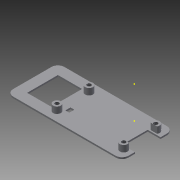
# Autodesk Inventor part: Case Relay
Saved by Autodesk Inventor 2015 (Build 190159000, 159)
## iProperties
Created: 2017-12-18
Part Number: Case Relay
Material: Generic
Document SubType Name: Modeling
Designer: Toby
Density: 1 g/cm^3
Appearance: Default
Author: Toby
Autodesk Inventor part; units mm, degrees
ref_plane "YZ Plane" through (0, 0, 0) normal (1, 0, 0) x (0, 1, 0)
ref_plane "XZ Plane" through (0, 0, 0) normal (0, 1, 0) x (-1, 0, 0)
ref_plane "XY Plane" through (0, 0, 0) normal (0, 0, 1) x (1, 0, 0)
sketch "Sketch1" plane through (0, 0, 0) normal (0, 0, 1) x (1, 0, 0)
  line L0 (-66.7657, 11.6667) -> (16.2343, 11.6667)
  line L1 (16.2343, 11.6667) -> (16.2343, -23.3333)
  line L2 (16.2343, -23.3333) -> (-66.7657, -23.3333)
  line L3 (-66.7657, -23.3333) -> (-66.7657, 11.6667)
  point P0 (0, 0)
  dimension "d0" = 35
  dimension "d1" = 83
  constraints: 8 end point, 2 parallel, 1 horizontal, 1 perpendicular
  measures "d0" distance of L2.end L0.start
  measures "d1" distance of L0.start L0.end
extrude "Extrusion1" add sketch "Sketch1" along normal blind 1.2
sketch "Sketch2" plane through (0, 0, 1.2) normal (0, 0, 1) x (1, 0, 0)
  line L0 (16.2343, -23.3333) -> (16.2343, 11.6667) projected
  line L1 (-66.7657, 11.6667) -> (16.2343, 11.6667)
  line L2 (16.2343, 11.6667) -> (16.2343, 9.8667)
  line L3 (16.2343, 9.8667) -> (-66.7657, 9.8667)
  line L4 (-66.7657, 9.8667) -> (-66.7657, 11.6667)
  line L5 (-66.7657, 11.6667) -> (-66.7657, -23.3333) projected
  line L6 (16.2343, -23.3333) -> (-66.7657, -23.3333)
  line L7 (-66.7657, -23.3333) -> (-66.7657, -21.5333)
  line L8 (-66.7657, -21.5333) -> (16.2343, -21.5333)
  line L9 (16.2343, -21.5333) -> (16.2343, -23.3333)
  line L10 (-66.7657, 9.8667) -> (-65.5657, 9.8667)
  line L11 (-65.5657, 9.8667) -> (-65.5657, -21.5333)
  line L12 (-65.5657, -21.5333) -> (-66.7657, -21.5333)
  line L13 (-66.7657, -21.5333) -> (-66.7657, 9.8667)
  line L14 (16.2343, 9.8667) -> (15.0343, 9.8667)
  line L15 (15.0343, 9.8667) -> (15.0343, -21.5333)
  line L16 (15.0343, -21.5333) -> (16.2343, -21.5333)
  line L17 (16.2343, -21.5333) -> (16.2343, 9.8667)
  line L18 (-66.7657, 11.6667) -> (-65.5657, 11.6667)
  line L19 (-65.5657, 11.6667) -> (-65.5657, -21.5333)
  line L20 (-65.5657, -21.5333) -> (-66.7657, -21.5333)
  line L21 (-66.7657, -21.5333) -> (-66.7657, 11.6667)
  line L22 (-66.7657, 11.6667) -> (16.2343, 11.6667)
  line L23 (16.2343, 11.6667) -> (16.2343, 9.8667)
  line L24 (16.2343, 9.8667) -> (-66.7657, 9.8667)
  line L25 (-66.7657, 9.8667) -> (-66.7657, 11.6667)
  point P0 (0, 0)
  dimension "d4" = 1.8
  dimension "d5" = 1.8
  dimension "d6" = 1.2
  dimension "d7" = 1.2
  constraints: 48 end point, 12 parallel, 6 horizontal, 6 perpendicular, 4 point on line
  measures "d4" distance between parallel lines of L1 L3
  measures "d5" distance between parallel lines of L6 L8
  measures "d6" distance between parallel lines of L13 L11
  measures "d7" distance between parallel lines of L17 L15
extrude "Extrusion2" add sketch "Sketch2" along normal blind 30 contours L6 L5 L8 L0 | L8 L15 L3 L0 | L3 L19 L1 L0 | L5 L3 L11 L8 | L4 L1 L19 L3
sketch "Sketch3" plane through (0, 0, 31.2) normal (0, 0, 1) x (1, 0, 0)
  point P0 (0, 0)
sketch "Sketch4" plane through (16.2343, -23.3333, 0) normal (1, 0, 0) x (0, 0, -1)
  line L0 (-1.2, 33.2) -> (-1.2, 1.8) projected
  line L1 (-1.2, 7.5) -> (-6.2, 7.5)
  line L2 (-6.2, 7.5) -> (-6.2, 27.5)
  line L3 (-6.2, 27.5) -> (-1.2, 27.5)
  line L4 (-1.2, 27.5) -> (-1.2, 7.5)
  line L5 (-1.2, 1.8) -> (-31.2, 1.8) projected
  line L6 (-1.2, 33.2) -> (-31.2, 33.2) projected
  line L7 (-6.2, 7.5) -> (0, 7.5)
  line L8 (0, 7.5) -> (0, 27.5)
  line L9 (0, 27.5) -> (-6.2, 27.5)
  line L10 (-6.2, 27.5) -> (-6.2, 7.5)
  line L11 (0, 35) -> (0, 0) projected
  point P0 (0, 23.3333)
  dimension "d10" = 20
  dimension "d11" = 5
  dimension "d12" = 5.7
  dimension "d13" = 5.7
  constraints: 16 end point, 4 parallel, 2 collinear, 2 horizontal, 2 perpendicular, 1 point on line
  measures "d10" distance of L1.end L2.end
  measures "d11" distance between parallel lines of L2 L0
  measures "d12" distance between parallel lines of L5 L1
  measures "d13" distance between parallel lines of L6 L3
extrude "Extrusion3" cut sketch "Sketch4" against normal blind 10
fillet "Fillet1" radius 2 8 edges at (-66.7657, 11.6667, 15.6) (-65.5657, 9.8667, 16.2) (-66.7657, -23.3333, 15.6) (-65.5657, -21.5333, 16.2) (15.0343, 9.8667, 16.2) (16.2343, 11.6667, 15.6) (16.2343, -23.3333, 15.6) (15.0343, -21.5333, 16.2)
sketch "Sketch5" plane through (0, 0, 1.2) normal (0, 0, 1) x (1, 0, 0)
  circle A0 centre (10.0343, 6.6667) radius 1.5
  circle A1 centre (10.0343, -18.3333) radius 1.5
  line L0 (15.0343, 7.8667) -> (15.0343, -19.5333) projected
  line L1 (13.0343, -21.5333) -> (-63.5657, -21.5333) projected
  line L2 (-63.5657, 9.8667) -> (13.0343, 9.8667) projected
  point P0 (0, 0)
  dimension "d17" = 3
  dimension "d18" = 3
  dimension "d19" = 25
  dimension "d20" = 5
  dimension "d21" = 5
  dimension "d22" = 3.2
  dimension "d23" = 3.2
  constraints: 2 centre point
  measures "d17" diameter of A0
  measures "d18" diameter of A1
  measures "d19" distance of A1.centre A0.centre
  measures "d20" distance from line of L0 A0.centre
  measures "d21" distance from line of L0 A1.centre
  measures "d22" distance from line of L1 A1.centre
  measures "d23" distance from line of L2 A0.centre
extrude "Extrusion4" add sketch "Sketch5" along normal blind 5
sketch "Sketch6" plane through (0, 0, 1.2) normal (0, 0, 1) x (1, 0, 0)
  circle A0 centre (-41.9656, -18.3962) radius 1.5
  circle A1 centre (-41.9656, 6.6038) radius 1.5
  circle A2 centre (10.0343, 6.6667) radius 1.5 projected
  circle A3 centre (10.0343, -18.3333) radius 1.5 projected
  point P0 (0, 0)
  dimension "d26" = 3
  dimension "d27" = 3
  dimension "d28" = 25
  dimension "d29" = 52
  dimension "d30" = 52
  constraints: 2 centre point
  measures "d26" diameter of A0
  measures "d27" diameter of A1
  measures "d28" distance of A1.centre A0.centre
  measures "d29" distance of A2.centre A1.centre
  measures "d30" distance of A3.centre A0.centre
extrude "Extrusion5" add sketch "Sketch6" along normal blind 5 contours A0 | A1
sketch "Sketch7" plane through (-41.9656, 6.6038, 6.2) normal (0, 0, 1) x (1, 0, 0)
  point P0 (41.9656, -6.6038)
sketch "Sketch8" plane through (0, 0, 1.2) normal (0, 0, 1) x (1, 0, 0)
  circle A0 centre (-41.9656, -18.3962) radius 1.5 projected
  circle A1 centre (-41.9656, -18.3962) radius 3
  circle A2 centre (-41.9656, 6.6038) radius 1.5 projected
  circle A3 centre (-41.9656, 6.6038) radius 3
  circle A4 centre (10.0343, -18.3333) radius 1.5 projected
  circle A5 centre (10.0343, -18.3333) radius 3
  circle A6 centre (10.0343, 6.6667) radius 1.5 projected
  circle A7 centre (10.0343, 6.6667) radius 3
  point P0 (0, 0)
  dimension "d33" = 6
  dimension "d34" = 6
  dimension "d35" = 6
  dimension "d36" = 6
  constraints: 4 centre point, 4 coincident
  measures "d33" diameter of A1
  measures "d34" diameter of A3
  measures "d35" diameter of A7
  measures "d36" diameter of A5
extrude "Extrusion6" add sketch "Sketch8" along normal blind 5
sketch "Sketch9" plane through (0, 0, 1.2) normal (0, 0, 1) x (1, 0, 0)
  arc A0 (8.376, -15.8333) -> (11.6926, -15.8333) centre (10.0343, -18.3333) ccw projected
  circle A1 centre (10.0343, -18.3333) radius 3
  arc A2 (11.6926, 4.1667) -> (8.376, 4.1667) centre (10.0343, 6.6667) ccw projected
  circle A3 centre (10.0343, 6.6667) radius 3
  point P0 (0, 0)
  dimension "d39" = 6
  dimension "d40" = 6
  constraints: 2 centre point, 2 coincident
  measures "d39" diameter of A1
  measures "d40" diameter of A3
extrude "Extrusion7" add sketch "Sketch9" against normal blind 1.2
sketch "Sketch10" plane through (-41.9656, -18.3962, 6.2) normal (0, 0, 1) x (1, 0, 0)
  circle A0 centre (0, 0) radius 3 projected
  circle A1 centre (0, 0) radius 1.5
  circle A2 centre (0, 25) radius 3 projected
  circle A3 centre (0, 25) radius 1.5
  circle A4 centre (52, 0.0629) radius 3 projected
  circle A5 centre (52, 0.0629) radius 1.5
  circle A6 centre (52, 25.0629) radius 3 projected
  circle A7 centre (52, 25.0629) radius 1.5
  point P0 (41.9656, 18.3962)
  dimension "d43" = 3
  dimension "d44" = 3
  dimension "d45" = 3
  dimension "d46" = 3
  constraints: 4 centre point, 4 coincident
  measures "d43" diameter of A1
  measures "d44" diameter of A3
  measures "d45" diameter of A5
  measures "d46" diameter of A7
extrude "Extrusion8" cut sketch "Sketch10" against normal blind 4 contours A1 | A3 | A5 | A7
thread "Thread1" size "M3x0.5" class "6H" standard "ANSI Metric M Profile" full length
thread "Thread2" size "M3x0.5" class "6H" standard "ANSI Metric M Profile" full length
thread "Thread3" size "M3x0.5" class "6H" standard "ANSI Metric M Profile" full length
thread "Thread4" size "M3x0.5" class "6H" standard "ANSI Metric M Profile" full length
sketch "Sketch11" plane through (0, 0, 31.2) normal (0, 0, 1) x (1, 0, 0)
  arc A0 (-64.7657, 11.6667) -> (-66.7657, 9.6667) centre (-64.7657, 9.6667) ccw projected
  line L0 (-66.7657, 9.6667) -> (16.2343, 9.6667)
  line L1 (16.2343, 9.6667) -> (16.2343, 14.6667)
  line L2 (16.2343, 14.6667) -> (-66.7657, 14.6667)
  line L3 (-66.7657, 14.6667) -> (-66.7657, 9.6667)
  line L4 (16.2343, -21.3333) -> (-66.7657, -21.3333)
  line L5 (-66.7657, -21.3333) -> (-66.7657, -26.3333)
  line L6 (-66.7657, -26.3333) -> (16.2343, -26.3333)
  line L7 (16.2343, -26.3333) -> (16.2343, -21.3333)
  point P0 (0, 0)
  dimension "d57" = 5
  dimension "d58" = 5
  dimension "d59" = 83
  constraints: 16 end point, 4 parallel, 2 horizontal, 2 perpendicular, 1 point on circle, 1 point on line
  measures "d57" distance of L1.end L0.end
  measures "d58" distance of L5.end L4.end
  measures "d59" distance between parallel lines of L3 L1
extrude "Extrusion9" add sketch "Sketch11" against normal blind 31.2
fillet "Fillet2" radius 2 4 edges at (16.2343, -26.3333, 15.6) (16.2343, 14.6667, 15.6) (-66.7657, 14.6667, 15.6) (-66.7657, -26.3333, 15.6)
sketch "Sketch12" plane through (0, 0, 31.2) normal (0, 0, 1) x (1, 0, 0)
  line L0 (14.2343, -26.3333) -> (-64.7657, -26.3333) projected
  line L1 (8.2343, -26.3333) -> (-58.7657, -26.3333)
  line L2 (-58.7657, -26.3333) -> (-58.7657, -23.1333)
  line L3 (-58.7657, -23.1333) -> (8.2343, -23.1333)
  line L4 (8.2343, -23.1333) -> (8.2343, -26.3333)
  line L5 (-64.7657, 14.6667) -> (14.2343, 14.6667) projected
  line L6 (8.2343, 14.6667) -> (-58.7657, 14.6667)
  line L7 (-58.7657, 14.6667) -> (-58.7657, 11.4667)
  line L8 (-58.7657, 11.4667) -> (8.2343, 11.4667)
  line L9 (8.2343, 11.4667) -> (8.2343, 14.6667)
  line L10 (16.2343, -24.3333) -> (16.2343, 12.6667) projected
  line L11 (-66.7657, 12.6667) -> (-66.7657, -24.3333) projected
  line L12 (13.9061, -21.3333) -> (-64.4375, -21.3333) projected
  line L13 (10.0343, 9.6667) -> (-64.4375, 9.6667) projected
  point P0 (0, 0)
  dimension "d63" = 8
  dimension "d64" = 8
  dimension "d65" = 1.8
  dimension "d66" = 1.8
  constraints: 16 end point, 4 parallel, 4 point on line, 2 horizontal, 2 perpendicular
  measures "d63" distance between parallel lines of L10 L4
  measures "d64" distance between parallel lines of L11 L2
  measures "d65" distance between parallel lines of L12 L3
  measures "d66" distance between parallel lines of L13 L8
extrude "Extrusion10" cut sketch "Sketch12" against normal blind 31.2
fillet "Fillet3" radius 2 4 edges at (8.2343, -26.3333, 15.6) (-58.7657, -26.3333, 15.6) (8.2343, 14.6667, 15.6) (-58.7657, 14.6667, 15.6)
sketch "Sketch13" plane through (0, 0, 31.2) normal (0, 0, 1) x (1, 0, 0)
  line L0 (14.2343, -26.3333) -> (10.2343, -26.3333) projected
  circle A0 centre (12.2343, -23.9333) radius 1.5
  circle A1 centre (-62.7657, -23.9333) radius 1.5
  line L1 (-64.7657, -26.3333) -> (-60.7657, -26.3333) projected
  circle A2 centre (12.2343, 12.2667) radius 1.5
  circle A3 centre (-62.7657, 12.2667) radius 1.5
  line L2 (-66.7657, 12.6667) -> (-66.7657, -24.3333) projected
  line L3 (-60.7657, 14.6667) -> (-64.7657, 14.6667) projected
  line L4 (16.2343, -24.3333) -> (16.2343, 12.6667) projected
  line L5 (14.2343, 14.6667) -> (10.2343, 14.6667) projected
  line L6 (8.2343, -23.1333) -> (8.2343, -24.3333) projected
  point P0 (0, 0)
  dimension "d70" = 2.4
  dimension "d71" = 3
  dimension "d72" = 3
  dimension "d73" = 2.4
  dimension "d74" = 3
  dimension "d75" = 3
  dimension "d76" = 4
  dimension "d77" = 4
  dimension "d78" = 2.4
  dimension "d79" = 4
  dimension "d80" = 2.4
  dimension "d81" = 4
  constraints: 4 centre point, 1 coincident
  measures "d70" distance from line of L0 point (12.234, -23.933)
  measures "d71" diameter of A0
  measures "d72" diameter of A1
  measures "d73" distance from line of A1.centre L1
  measures "d74" diameter of A2
  measures "d75" diameter of A3
  measures "d76" distance from line of L2 A1.centre
  measures "d77" distance from line of L2 A3.centre
  measures "d78" distance from line of L3 A3.centre
  measures "d79" distance from line of L4 A2.centre
  measures "d80" distance from line of L5 A2.centre
  measures "d81" distance from line of L6 A0.centre
hole "Hole1" at (12.2343, -23.9333, 31.2) at (12.2343, 12.2667, 31.2) at (-62.7657, -23.9333, 31.2) at (-62.7657, 12.2667, 31.2) direction (0, 0, -1) diameter 3 depth 5 tip angle 118
sketch "Sketch14" plane through (0, 0, 31.2) normal (0, 0, 1) x (1, 0, 0)
  line L0 (-68.9331, 15.611) -> (20.031, 15.611)
  line L1 (20.031, 15.611) -> (20.031, -27.6485)
  line L2 (20.031, -27.6485) -> (-68.9331, -27.6485)
  line L3 (-68.9331, -27.6485) -> (-68.9331, 15.611)
  point P0 (0, 0)
  constraints: 8 end point, 2 parallel, 1 horizontal, 1 perpendicular
extrude "Extrusion11" cut sketch "Sketch14" against normal blind 25
sketch "Sketch15" plane through (0, 0, 6.2) normal (0, 0, 1) x (1, 0, 0)
  line L0 (-73.259, 21.6297) -> (22.194, 21.6297)
  line L1 (22.194, 21.6297) -> (22.194, 9.6667)
  line L2 (22.194, 9.6667) -> (-73.259, 9.6667)
  line L3 (-73.259, 9.6667) -> (-73.259, 21.6297)
  line L4 (-69.8735, -21.3333) -> (26.0497, -21.3333)
  line L5 (26.0497, -21.3333) -> (26.0497, -30.3757)
  line L6 (26.0497, -30.3757) -> (-69.8735, -30.3757)
  line L7 (-69.8735, -30.3757) -> (-69.8735, -21.3333)
  line L8 (10.0343, 9.6667) -> (-64.4375, 9.6667) projected
  line L9 (-41.3548, -21.3333) -> (10.0343, -21.3333) projected
  point P0 (0, 0)
  constraints: 16 end point, 4 parallel, 2 collinear, 2 horizontal, 2 perpendicular
extrude "Extrusion12" cut sketch "Sketch15" against normal blind 25
sketch "Sketch16" plane through (0, 0, 1.2) normal (0, 0, 1) x (1, 0, 0)
  line L0 (6.2343, 4.1667) -> (16.2343, 4.1667)
  line L1 (16.2343, 4.1667) -> (16.2343, -15.8333)
  line L2 (16.2343, -15.8333) -> (6.2343, -15.8333)
  line L3 (6.2343, -15.8333) -> (6.2343, 4.1667)
  point P0 (0, 0)
  constraints: 8 end point, 2 parallel, 1 horizontal, 1 perpendicular
extrude "Extrusion13" cut sketch "Sketch16" against normal blind 25
sketch "Sketch17" plane through (0, 0, 1.2) normal (0, 0, 1) x (1, 0, 0)
  line L0 (6.2343, 4.1667) -> (16.2343, 4.1667)
  line L1 (16.2343, 4.1667) -> (16.2343, -15.8333)
  line L2 (16.2343, -15.8333) -> (6.2343, -15.8333)
  line L3 (6.2343, -15.8333) -> (6.2343, 4.1667)
  point P0 (0, 0)
  constraints: 8 end point, 2 parallel, 1 horizontal, 1 perpendicular
extrude "Extrusion14" cut sketch "Sketch17" along normal blind 25
sketch "Sketch18" plane through (0, 0, 1.2) normal (0, 0, 1) x (1, 0, 0)
  line L0 (15.0343, -19.5333) -> (15.0343, -15.8333) projected
  line L1 (6.2343, 5.1667) -> (15.0343, 5.1667)
  line L2 (15.0343, 5.1667) -> (15.0343, -16.8333)
  line L3 (15.0343, -16.8333) -> (6.2343, -16.8333)
  line L4 (6.2343, -16.8333) -> (6.2343, 5.1667)
  line L5 (6.2343, 4.1667) -> (8.376, 4.1667) projected
  line L6 (15.0343, -15.8333) -> (11.6926, -15.8333) projected
  line L7 (6.2343, -15.8333) -> (6.2343, 4.1667) projected
  point P0 (0, 0)
  dimension "d97" = 1
  dimension "d98" = 1
  constraints: 8 end point, 2 parallel, 1 collinear, 1 horizontal, 1 perpendicular, 1 point on line
  measures "d97" distance between parallel lines of L5 L1
  measures "d98" distance between parallel lines of L6 L3
extrude "Extrusion15" cut sketch "Sketch18" along normal blind 25
sketch "Sketch19" plane through (0, 0, 6.2) normal (0, 0, 1) x (1, 0, 0)
  line L0 (13.9061, 9.6667) -> (16.2343, 9.6667)
  line L1 (16.2343, 9.6667) -> (16.2343, -21.3333)
  line L2 (16.2343, -21.3333) -> (13.9061, -21.3333)
  line L3 (13.9061, -21.3333) -> (13.9061, 9.6667)
  line L4 (-66.7657, 9.6667) -> (-64.4375, 9.6667)
  line L5 (-64.4375, 9.6667) -> (-64.4375, -21.3333)
  line L6 (-64.4375, -21.3333) -> (-66.7657, -21.3333)
  line L7 (-66.7657, -21.3333) -> (-66.7657, 9.6667)
  point P0 (0, 0)
  constraints: 16 end point, 4 parallel, 2 horizontal, 2 perpendicular
extrude "Extrusion16" cut sketch "Sketch19" against normal blind 5
sketch "Sketch20" plane through (0, 0, 1.2) normal (0, 0, 1) x (1, 0, 0)
  line L0 (-73.7657, 14.1667) -> (16.2343, 14.1667)
  line L1 (16.2343, 14.1667) -> (16.2343, -25.8333)
  line L2 (16.2343, -25.8333) -> (-73.7657, -25.8333)
  line L3 (-73.7657, -25.8333) -> (-73.7657, 14.1667)
  line L4 (16.2343, 9.6667) -> (16.2343, 4.1667) projected
  line L5 (-66.7657, 9.6667) -> (16.2343, 9.6667) projected
  line L6 (-41.3548, -21.3333) -> (10.0343, -21.3333) projected
  line L7 (-66.7657, -21.3333) -> (-66.7657, 9.6667) projected
  line L8 (16.2343, 4.1667) -> (6.2343, 4.1667)
  line L9 (6.2343, 4.1667) -> (6.2343, -15.8333)
  line L10 (6.2343, -15.8333) -> (16.2343, -15.8333)
  line L11 (16.2343, -15.8333) -> (16.2343, 4.1667)
  point P0 (0, 0)
  dimension "d103" = 90
  dimension "d104" = 40
  dimension "d105" = 4.5
  dimension "d106" = 4.5
  dimension "d107" = 7
  constraints: 16 end point, 4 parallel, 2 horizontal, 2 perpendicular, 1 collinear
  measures "d103" distance between parallel lines of L1 L3
  measures "d104" distance between parallel lines of L2 L0
  measures "d105" distance between parallel lines of L5 L0
  measures "d106" distance between parallel lines of L2 L6
  measures "d107" distance between parallel lines of L3 L7
extrude "Extrusion17" add sketch "Sketch20" against normal blind 1.2 contours L0 L1 L8 L9 L10 L2 L3
fillet "Fillet4" radius 5 4 edges at (-73.7657, 14.1667, 0.6) (-73.7657, -25.8333, 0.6) (16.2343, -25.8333, 0.6) (16.2343, 14.1667, 0.6)
sketch "Sketch21" plane through (0, 0, 1.2) normal (0, 0, 1) x (1, 0, 0)
  line L0 (-65.7657, 6.1667) -> (-46.9656, 6.1667)
  line L1 (-46.9656, 6.1667) -> (-46.9656, -17.8333)
  line L2 (-46.9656, -17.8333) -> (-65.7657, -17.8333)
  line L3 (-65.7657, -17.8333) -> (-65.7657, 6.1667)
  line L4 (-68.7657, 14.1667) -> (11.2343, 14.1667) projected
  line L5 (11.2343, -25.8333) -> (-68.7657, -25.8333) projected
  line L6 (-73.7657, -20.8333) -> (-73.7657, 9.1667) projected
  circle A0 centre (-41.9656, 6.6038) radius 1.5 projected
  point P0 (0, 0)
  dimension "d111" = 8
  dimension "d112" = 8
  dimension "d113" = 8
  dimension "d114" = 5
  constraints: 8 end point, 2 parallel, 1 horizontal, 1 perpendicular
  measures "d111" distance between parallel lines of L4 L0
  measures "d112" distance between parallel lines of L5 L2
  measures "d113" distance between parallel lines of L6 L3
  measures "d114" distance from line of A0.centre L1
extrude "Extrusion18" cut sketch "Sketch21" against normal blind 1.2 contours L0 L1 L2 L3
sketch "Sketch22" plane through (0, 0, 1.2) normal (0, 0, 1) x (1, 0, 0)
  line L0 (-38.9656, -10.8333) -> (-35.9656, -10.8333)
  line L1 (-35.9656, -10.8333) -> (-35.9656, -14.8333)
  line L2 (-35.9656, -14.8333) -> (-38.9656, -14.8333)
  line L3 (-38.9656, -14.8333) -> (-38.9656, -10.8333)
  line L4 (-46.9656, -17.8333) -> (-65.7657, -17.8333) projected
  circle A0 centre (-41.9656, -18.3962) radius 1.5 projected
  line L5 (11.2343, -25.8333) -> (-68.7657, -25.8333) projected
  point P0 (0, 0)
  dimension "d117" = 3
  dimension "d119" = 4
  dimension "d120" = 3
  dimension "d121" = 11
  constraints: 8 end point, 2 parallel, 1 horizontal, 1 perpendicular
  measures "d117" distance between parallel lines of L3 L1
  measures "d119" distance of L2.end L0.start
  measures "d120" distance from line of A0.centre L3
  measures "d121" distance between parallel lines of L5 L2
extrude "Extrusion19" cut sketch "Sketch22" against normal blind 1.2 contours L0 L1 L2 L3
body "Solid1"
